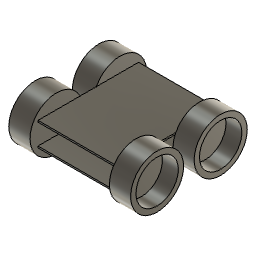
XLR8 Bot v1 (Autodesk Fusion 360 design; units mm, degrees)
Autodesk Fusion 360 part; units mm, degrees
sketch "Sketch1" plane through (0, 0, 0) normal (0, 0, 1) x (1, 0, 0)
  line L0 (75, -95) -> (-75, -95)
  line L1 (-75, -95) -> (-75, 95)
  line L2 (-75, 95) -> (75, 95)
  line L3 (75, 95) -> (75, -95)
  line L4 (75, -95) -> (-75, 95) construction
  line L5 (-75, -95) -> (75, 95) construction
  dimension "d1" = 150
  dimension "d2" = 190
  constraint horizontal L0
  constraint perpendicular L0 L1
  constraint parallel L0 L2
  constraint parallel L1 L3
  constraint coincident L4 origin
  constraint coincident L5 origin
  measures "d1" distance of L1.end L2.end
  measures "d2" distance of L0.end L1.end
ref_plane "WorkPlane1" through (0, 0, 45) normal (0, 0, 1) x (1, 0, 0)
sketch "Sketch2" plane through (0, 0, 45) normal (0, 0, 1) x (1, 0, 0)
  line L0 (75, -95) -> (-75, -95)
  line L1 (-75, -95) -> (-75, 95)
  line L2 (-75, 95) -> (75, 95)
  line L3 (75, 95) -> (75, -95)
  line L4 (75, -95) -> (-75, 95) construction
  line L5 (-75, -95) -> (75, 95) construction
  dimension "d4" = 150
  dimension "d5" = 190
  constraint horizontal L0
  constraint perpendicular L0 L1
  constraint parallel L0 L2
  constraint parallel L1 L3
  constraint coincident L4 origin
  constraint coincident L5 origin
  measures "d4" distance of L1.end L2.end
  measures "d5" distance of L0.end L1.end
sketch "Sketch3" plane through (0, 0, 45) normal (0, 0, 1) x (1, 0, 0)
ref_plane "WorkPlane2" through (75, 95, 45) normal (-1, 0, 0) x (0, -1, 0)
sketch "Sketch4" plane through (75, 95, 45) normal (-1, 0, 0) x (0, -1, 0)
  circle A0 centre (155, -22.5) radius 50
  line L0 (0, 0) -> (190, 0)
  circle A1 centre (35, -22.5) radius 50
  dimension "d6" = 100
  dimension "d7" = 22.5
  dimension "d8" = 100
  dimension "d9" = 22.5
  dimension "d10" = 120
  dimension "d11" = 155
  measures "d6" diameter of A0
  measures "d7" distance of A0.centre L0
  measures "d8" diameter of A1
  measures "d9" distance of L0 A1.centre
  measures "d10" distance of A0.centre A1.centre
  measures "d11" horizontal distance of L0.start A0.centre
ref_plane "WorkPlane3" through (-75, -95, 45) normal (1, 0, 0) x (0, 1, 0)
sketch "Sketch5" plane through (-75, -95, 45) normal (1, 0, 0) x (0, 1, 0)
  circle A0 centre (155, -22.5) radius 50
  circle A1 centre (35, -22.5) radius 50
  line L0 (0, 0) -> (190, 0)
  dimension "d12" = 100
  dimension "d13" = 100
  dimension "d14" = 120
  dimension "d15" = 155
  dimension "d16" = 22.5
  dimension "d17" = 22.5
  measures "d12" diameter of A0
  measures "d13" diameter of A1
  measures "d14" distance of A0.centre A1.centre
  measures "d15" horizontal distance of A0.centre L0.start
  measures "d16" distance of A0.centre L0
  measures "d17" distance of A1.centre L0
extrude "Extrude1" add sketch "Sketch2" against normal blind 3 makes body 1
extrude "Extrude2" add sketch "Sketch1" along normal blind 3 separate body makes body 2
extrude "Extrude3" add sketch "Sketch4" against normal blind 40 bodies 1 2
extrude "Extrude4" add sketch "Sketch5" against normal blind 40 bodies 1
sketch "Sketch6" plane through (115, 0, 0) normal (1, 0, 0) x (0, 1, 0)
  circle A0 centre (-60, 22.5) radius 50
  circle A1 centre (-60, 22.5) radius 40
  dimension "d26" = -10
sketch "Sketch7" plane through (115, 0, 0) normal (1, 0, 0) x (0, 1, 0)
  circle A0 centre (60, 22.5) radius 50
  circle A1 centre (60, 22.5) radius 40
  dimension "d27" = -10
extrude "Extrude5" cut sketch "Sketch6" sketch "Sketch7" against normal blind 30 contours A1 of sketch 2 contours A1 bodies 1
sketch "Sketch8" plane through (-115, 0, 0) normal (-1, 0, 0) x (0, -1, 0)
  circle A0 centre (-60, 22.5) radius 50
  circle A1 centre (-60, 22.5) radius 40
  dimension "d30" = -10
sketch "Sketch9" plane through (-115, 0, 0) normal (-1, 0, 0) x (0, -1, 0)
  circle A0 centre (60, 22.5) radius 50
  circle A1 centre (60, 22.5) radius 40
  dimension "d31" = -10
extrude "Extrude6" cut sketch "Sketch8" sketch "Sketch9" against normal blind 30 contours A1 of sketch 2 contours A1 bodies 1
